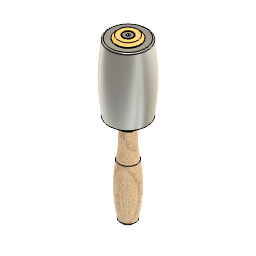
model (Autodesk Fusion 360 design; units mm, degrees)
Autodesk Fusion 360 part; units mm, degrees
sketch "side" plane through (0, 0, 0) normal (0, 1, 0) x (1, 0, 0)
  line L0 (0, 0) -> (0, -98)
  line L1 (0, -98) -> (27, -98) construction
  arc A0 (27, -98) -> (27, 0) centre (-271.125, -49) ccw
  line L2 (27, 0) -> (0, 0) construction
  arc A1 (27, -98) -> (0, -97) centre (0, -462) ccw
  line L3 (0, -97) -> (27.1626, -97) construction
  line L4 (31, -49) -> (0, -49) construction
  arc A2 (0, -1) -> (27, 0) centre (0, 364) ccw
  line L5 (17.25, -97.4078) -> (17.25, -98.4078)
  line L6 (17.25, -98.4078) -> (13.75, -101.9078)
  line L7 (13.75, -101.9078) -> (0, -101.9078)
  line L8 (0, -101.9078) -> (0, -98)
  line L9 (17.25, -0.5922) -> (17.25, 0.4078)
  line L10 (17.25, 0.4078) -> (13.75, 3.9078)
  line L11 (13.75, 3.9078) -> (0, 3.9078)
  line L12 (0, 3.9078) -> (0, 0)
  arc A3 (10.1202, 11.9078) -> (11.5, 3.9078) centre (40.1017, 12.9601) ccw
  arc A4 (12.8587, 52.6343) -> (10.1202, 11.9078) centre (209.9971, 18.9227) ccw
  arc A5 (12.8587, 52.6343) -> (11, 126.0743) centre (-174.3082, 84.6407) ccw
  arc A6 (11, 126.0743) -> (7.8849, 129.123) centre (7.0964, 125.2015) ccw
  arc A7 (7.8849, 129.123) -> (0, 129.9078) centre (0, 89.9078) ccw
  line L13 (0, 129.9078) -> (0, 3.9078)
  point P0 (31, -49)
  point P1 (15.5, 90)
  point P2 (10, 20)
  dimension "d1" = 27
  dimension "d2" = 31
  dimension "d3" = 98
  dimension "d4" = 1
  dimension "d5" = 1
  dimension "d6" = 45
  dimension "d7" = 4.5
  dimension "d8" = 17.25
  dimension "d9" = 11.5
  dimension "d10" = 126
  dimension "d11" = 40
  dimension "d12" = 4
  dimension "d13" = 11
  dimension "d15" = 30
  dimension "d17" = 200
  dimension "d18" = 8
  dimension "d19" = 90
  dimension "d20" = 15.5
  dimension "d21" = 10
  dimension "d22" = 20
  constraint coincident L0.start L2.end
  constraint vertical L0
  constraint horizontal L2
  constraint coincident A0 P0
  constraint midpoint A0 P0
  constraint coincident L0 A1.end
  constraint coincident A0 L3.end
  constraint horizontal L3
  constraint horizontal L1
  constraint equal L1 L2
  constraint tangent A1 L3
  constraint coincident P0 L4.start
  constraint midpoint L0 L4.end
  constraint symmetric L1.end L4 A0.end
  constraint symmetric A1.end L4 A2.start
  constraint symmetric A1 L4 A2
  constraint vertical L5
  constraint vertical L8
  constraint horizontal L7
  constraint coincident A1 L5.start
  constraint symmetric L0.end L4 L0.start
  constraint symmetric L4 L5.start L9.start
  constraint symmetric L4 L5.end L9.end
  constraint symmetric L4 L6.end L10.end
  constraint symmetric L4 L7.end L11.end
  constraint coincident L11 A3.end
  constraint tangent A3 A4
  constraint tangent A4 A5
  constraint vertical L13
  constraint coincident A7.centre L13
  constraint tangent A6 A7
  constraint tangent A5 A6
  constraint coincident A5 P1
  constraint coincident A4 P2
  measures "d1" distance of L0.end L1.end
  measures "d2" horizontal distance of L0.end P0
  measures "d3" distance of L1.end A0.end
  measures "d4" vertical distance of L1.end L3.end
  measures "d5" distance of L5.start L5.end
  measures "d6" angle of L1 L6
  measures "d7" vertical distance of L5.start L6.end
  measures "d8" horizontal distance of L0.end L5.end
  measures "d9" distance of L11.end A3.end
  measures "d10" vertical distance of L11.end A7.end
  measures "d11" radius of A7
  measures "d12" radius of A6
  measures "d13" horizontal distance of A5.end A7.end
  measures "d15" radius of A3
  measures "d17" radius of A4
  measures "d18" vertical distance of A3.end A3.start
  measures "d19" vertical distance of A0.end P1
  measures "d20" horizontal distance of A7.end P1
  measures "d21" distance of L13 P2
  measures "d22" vertical distance of A0.end P2
revolve "Revolve1" add sketch "side" angle 360 about axis through (0, 0, 1.75) along (0, 0, 1) contours L0 A2 L9 L10 L11 L12 | L0 A1 L5 L6 L7 L8 makes body 1 at (6.5439, 3.9989, 97.0806) makes body 2 at (6.5439, 3.9989, 0.9194)
revolve "Revolve2" add sketch "side" angle 360 about axis through (0, 0, 1.75) along (0, 0, 1) separate body contours L0 A0 A1 A2 | L11 A3 A4 A5 A6 A7 L13 makes body 3 at (-30.9809, 0.1335, 45.6244) makes body 4 at (13.8909, 6.4073, -94.9168)
fillet "Fillet1" radius 2 2 edges at (-25.1728, -9.7636, 98) (-25.1728, -9.7636, 0) on bodies 3
sketch "top" plane through (0, 0, 101.9078) normal (0, 0, 1) x (-1, 0, 0)
  circle A0 centre (0, 0) radius 13.75
  circle A1 centre (0, 0) radius 6.25
  line L0 (-2.2914, 0) -> (-1.1457, -1.9844)
  line L1 (-1.1457, -1.9844) -> (1.1457, -1.9844)
  line L2 (1.1457, -1.9844) -> (2.2914, 0)
  line L3 (2.2914, 0) -> (1.1457, 1.9844)
  line L4 (1.1457, 1.9844) -> (-1.1457, 1.9844)
  line L5 (-1.1457, 1.9844) -> (-2.2914, 0)
  dimension "d27" = 12.5
  dimension "d28" = 3.9688
  constraint coincident A0.centre A1.centre
  constraint horizontal L1
  measures "d27" diameter of A1
  measures "d28" distance of L0.end L4.end
extrude "Extrude1" cut sketch "top" against normal blind 5 contours A1 | L0 L1 L2 L3 L4 L5 bodies 1 3
extrude "Extrude2" add sketch "top" against normal blind 5 separate body contours A1 | L0 L1 L2 L3 L4 L5 makes body 5
extrude "Extrude3" cut sketch "top" against normal blind 4 contours L0 L1 L2 L3 L4 L5 bodies 5
chamfer "Chamfer1" distance 1 angle 45 1 edges at (5.827, -2.2601, 101.9078) on bodies 1
equation "d1 = ( 54 / 2 ) * 1 mm"
equation "d2 = ( 62 / 2 ) * 1 mm"
equation "d8 = ( 34.5 / 2 ) * 1 mm"
equation "d9 = ( 23 / 2 ) * 1 mm"
equation "d20 = ( 31 / 2 ) * 1 mm"
equation "d28 = 5/32\""
